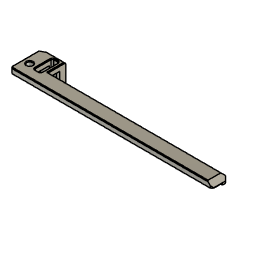
Bed_Fan_Wiring_Cover (Autodesk Fusion 360 design; units mm, degrees)
Autodesk Fusion 360 part; units mm, degrees
sketch "Sketch1" plane through (0, 0, 0) normal (0, 0, 1) x (1, 0, 0)
  line L0 (0, 0) -> (120, 0)
  line L1 (120, 0) -> (120, 10)
  line L2 (120, 10) -> (14, 10)
  line L3 (12, 15.4) -> (12, 6)
  line L4 (12, 6) -> (8, 6)
  line L5 (8, 6) -> (8, 17)
  line L6 (8, 17) -> (12, 17)
  line L7 (12, 17) -> (12, 15.4)
  line L8 (12, 15.4) -> (14, 15.4)
  line L9 (14, 15.4) -> (14, 20)
  line L10 (14, 20) -> (0, 20)
  line L11 (0, 20) -> (0, 0)
  line L12 (0, 7.5) -> (120, 7.5) construction
  circle A0 centre (4, 7.5) radius 1.7
  circle A1 centre (4, 7.5) radius 4 construction
  line L13 (0, 15) -> (8, 15) construction
  line L14 (0, 15.2) -> (8, 15.2)
  line L15 (14, 10) -> (14, 15.4)
  dimension "d1" = 120
  dimension "d2" = 10
  dimension "d3" = 7.5
  dimension "d4" = 3.4
  dimension "d5" = 8
  dimension "d6" = 1.5
  dimension "d7" = 4
  dimension "d8" = 2
  dimension "d9" = 3
  dimension "d11" = 2
  dimension "d12" = 4
  dimension "d13" = 0.4
  dimension "d14" = -0.2
  constraint coincident L0.start L11.end
  constraint horizontal L0
  constraint perpendicular L0 L1
  constraint perpendicular L1 L2
  constraint perpendicular L0 L3
  constraint perpendicular L1 L4
  constraint perpendicular L4 L5
  constraint perpendicular L1 L6
  constraint perpendicular L6 L7
  constraint perpendicular L6 L9
  constraint perpendicular L9 L10
  constraint perpendicular L0 L11
  constraint coincident L11 L12.start
  constraint coincident L1 L12.end
  constraint perpendicular L1 L12
  constraint coincident L12 A0.centre
  constraint concentric A0 A1
  constraint tangent L11 A1
  constraint tangent L5 A1
  constraint coincident L11 L13.start
  constraint coincident L5 L13.end
  constraint perpendicular L5 L13
  constraint perpendicular L7 L8
  constraint coincident L5 L14.end
  constraint coincident L11 L14.start
  constraint coincident L3.start L7.end
  constraint perpendicular L2 L15
  measures "d1" distance of L0.start L0.end
  measures "d2" distance of L0.end L1.end
  measures "d3" distance of L0 L12
  measures "d4" diameter of A0
  measures "d5" diameter of A1
  measures "d6" distance of L4 L12
  measures "d7" distance of L3.end L4.end
  measures "d8" distance of L6 L13
  measures "d9" distance of L6 L10
  measures "d11" distance of L3.start L8.end
  measures "d12" distance of L5.end L6.end
  measures "d13" distance of L8 L13
extrude "Extrude1" add sketch "Sketch1" against normal blind 3 contours L0 L1 L2 L3 L4 L5 L8 L11 L14 L15
extrude "Extrude2" add sketch "Sketch1" against normal up to surface (13 mm away) contours L5 L6 L7 L8 L9 L10 L11 L14
chamfer "Chamfer1" distance 1 angle 45 2 edges at (0, 0, -1.5) (120, 0, -1.5)
chamfer "Chamfer2" distance 2 angle 45 1 edges at (120, 10, -1.5)
chamfer "Chamfer3" distance 1 angle 45 1 edges at (12, 10.7, -3)
chamfer "Chamfer4" distance 8 distance2 6 1 edges at (0, 17.6, -13) measured on face at (0, 18.4, -5.3333)
chamfer "Chamfer5" distance 1.8 angle 45 2 edges at (7, 20, 0) (10, 20, -13)
chamfer "Chamfer6" distance 2.8 angle 45 1 edges at (120, 4.5, 0)
chamfer "Chamfer7" distance 2 angle 45 1 edges at (65.6, 10, 0)
chamfer "Chamfer8" distance 3 distance2 6 1 edges at (0, 20, -3.4) measured on face at (0, 11.4667, -1)
chamfer "Chamfer9" distance 1 angle 45 1 edges at (14, 20, -6.5)
fillet "Fillet1" radius 0.8 4 edges at (12, 6, -1) (8, 6, -1.5) (8, 17, -6.5) (12, 17, -6.5)
chamfer "Chamfer10" distance 0.4 angle 45 14 edges at (59.1, 0, 0) (0.5, 0.5, 0) (0, 9, 0) (2.415, 8.1147, 0) (8.2343, 6.2343, 0) (10, 6, 0) (11.7657, 6.2343, 0) (12, 11.5, 0) (11.7657, 16.7657, 0) (10, 17, 0) (8.2343, 16.7657, 0) (8, 11.5, 0) (14, 13.1, 0) (1.2, 17.6, 0)
sketch "Sketch2" plane through (0, 0, -3) normal (0, 0, -1) x (1, 0, 0)
  line L0 (13, -6) -> (13, -15.4)
  line L1 (13, -15.4) -> (14, -15.4)
  line L2 (14, -15.4) -> (14, -10)
  line L3 (14, -10) -> (118, -10)
  line L4 (118, -10) -> (120, -8)
  line L5 (120, -8) -> (120, -1)
  line L6 (120, -1) -> (119, 0)
  line L7 (119, 0) -> (1, 0)
  line L8 (1, 0) -> (0, -1)
  line L9 (0, -1) -> (0, -15.2)
  line L10 (0, -15.2) -> (8, -15.2)
  line L11 (8, -15.2) -> (8, -6.8)
  arc A0 (8.8, -6) -> (8, -6.8) centre (8.8, -6.8) ccw
  line L12 (8.8, -6) -> (13, -6)
  circle A1 centre (4, -7.5) radius 1.7
  line L13 (4, -7.5) -> (13, -7.5) construction
  line L14 (13, -7.5) -> (120, -7.5)
  constraint coincident A1.centre L13.start
  constraint perpendicular L5 L13
  constraint coincident L0 L13.end
  constraint coincident L5 L14.end
  constraint perpendicular L5 L14
extrude "Extrude3" add sketch "Sketch2" along normal blind 1 thin wall 3 centred open curves L14
delete_face "DeleteFace1" 1 faces at (119.6667, 8.6667, -3)
chamfer "Chamfer11" distance 1 angle 45 1 edges at (13, 7.5, -4)
chamfer "Chamfer12" distance 0.2 angle 45 2 edges at (66.5, 9, -4) (67, 6, -4)
